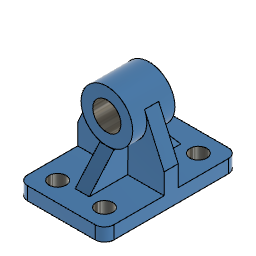
Figure-5 (Autodesk Fusion 360 design; units mm, degrees)
Autodesk Fusion 360 part; units mm, degrees
sketch "Sketch1" plane through (0, 0, 0) normal (0, 0, 1) x (1, 0, 0)
  line L0 (-46, 71) -> (46, 71)
  line L1 (46, 71) -> (46, -71)
  line L2 (46, -71) -> (-46, -71)
  line L3 (-46, -71) -> (-46, 71)
  line L4 (-46, 71) -> (46, -71) construction
  line L5 (46, 71) -> (-46, -71) construction
  dimension "d1" = 92
  dimension "d2" = 142
  constraint horizontal L0
  constraint perpendicular L0 L1
  constraint parallel L0 L2
  constraint parallel L1 L3
  constraint coincident L4 origin
  constraint coincident L5 origin
  measures "d1" distance of L1.end L2.end
  measures "d2" distance of L0.end L1.end
extrude "Extrude1" add sketch "Sketch1" along normal blind 14 makes body 1
fillet "Fillet1" radius 10 4 edges at (-46, -71, 7) (-46, 71, 7) (46, 71, 7) (46, -71, 7) on bodies 1
sketch "Sketch2" plane through (0, 0, 14) normal (0, 0, 1) x (-1, 0, 0)
  arc A0 (-36, 71) -> (-46, 61) centre (-36, 61) ccw
  line L0 (-46, 61) -> (-46, -61)
  arc A1 (-46, -61) -> (-36, -71) centre (-36, -61) ccw
  line L1 (-36, -71) -> (36, -71)
  arc A2 (36, -71) -> (46, -61) centre (36, -61) ccw
  line L2 (46, -61) -> (46, 61)
  arc A3 (46, 61) -> (36, 71) centre (36, 61) ccw
  line L3 (36, 71) -> (-36, 71)
  circle A4 centre (-25, 50) radius 9
  dimension "d7" = 18
  dimension "d8" = 21
  dimension "d9" = 21
  measures "d7" diameter of A4
  measures "d8" distance of L3 A4.centre
  measures "d9" distance of L0 A4.centre
extrude "Extrude2" cut sketch "Sketch2" against normal through all contours A4 bodies 1
pattern_linear "R-Pattern1" count 2 spacing 100 along (0, 1, 0) count 2 spacing 50 along (-1, 0, 0) of "Extrude2"
sketch "Sketch3" plane through (0, 0, 0) normal (0, 1, 0) x (1, 0, 0)
  circle A0 centre (0, -72) radius 15
  circle A1 centre (0, -72) radius 27.5
  line L0 (36, -14) -> (-36, -14)
  dimension "d16" = 30
  dimension "d17" = 55
  constraint concentric A0 A1
  measures "d16" diameter of A0
  measures "d17" diameter of A1
extrude "Extrude3" add sketch "Sketch3" along normal mid plane 45 separate body makes body 2
sketch "Sketch4" plane through (0, 0, 0) normal (0, 1, 0) x (1, 0, 0)
  line L0 (-46, -14) -> (-46, -36)
  line L1 (-46, -36) -> (-25.1484, -83.127)
  line L2 (-25.1484, -83.127) -> (-25.1483, -83.127)
  arc A0 (-25.1483, -83.127) -> (25.1484, -83.127) centre (0, -72) ccw
  line L3 (46, -36) -> (46, -14)
  line L4 (46, -14) -> (-46, -14)
  line L5 (25.1484, -83.127) -> (46, -36)
  circle A1 centre (0, -72) radius 27.5
  point P0 (46, -14)
  point P1 (-46, -14)
  dimension "d21" = 22
  constraint vertical L0
  constraint parallel L1 L2
  constraint tangent L2 A0
  constraint parallel L0 L3
  constraint equal L0 L3
  constraint coincident P0 L3.end
  constraint coincident P1 L0.start
  constraint concentric A0 A1
  constraint tangent L5 A1
  constraint tangent L1 A1
  constraint equal L1 L5
  measures "d21" distance of L3.start P0
extrude "Extrude4" add sketch "Sketch4" along normal mid plane 15 contours L0 L1 L3 L4 L5 A1 bodies 1 2
sketch "Sketch5" plane through (0, 0, 0) normal (1, 0, 0) x (0, 1, 0)
  line L0 (-7.7437, 14.4207) -> (-48.7437, 14.4207)
  line L1 (-22.5, 44.5) -> (-48.7437, 14.4207)
  line L2 (-22.5, 99.5) -> (-22.5, 44.5)
  arc A0 through (-7.5, 83.127, 25.1484) (-7.5, 44.5, 0) (-7.5, 83.127, -25.1484)
  line L3 (-7.7437, 14.4207) -> (-7.5, 44.5)
  line L4 (-7.5, 44.5) -> (-22.5, 44.5)
  dimension "d24" = 41
  constraint horizontal L0
  constraint coincident L1.start L2
  constraint coincident L1.start L2.end
  constraint coincident L0.end L1.end
  measures "d24" distance of L0.start L0.end
extrude "Extrude5" add sketch "Sketch5" along normal mid plane 15 separate body makes body 3
mirror "Mirror1" about plane through (0, 0, 0) normal (0, 1, 0) of bodies 3 makes body 4
